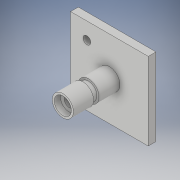
# Autodesk Inventor part: pieza_2_vinculacion
Saved by Autodesk Inventor 2019 (Build 230136000, 136)
## iProperties
Created: 2020-01-09
Part Number: pieza_2_vinculacion
Material: Generic
Document SubType Name: Modeling
Designer: Laptop
Density: 1 g/cm^3
Appearance: Default
Author: Laptop
## iProperties of the stored document pieza_2_vinculacion_3DPrint.ipt
Created: 2020-01-12
Part Number: pieza_2_vinculacion_3DPrint
Material: Generic
Document SubType Name: Modeling
Designer: Laptop
Density: 1 g/cm^3
Appearance: Default
Author: Laptop
Autodesk Inventor part; units mm, degrees
ref_plane "YZ Plane" through (0, 0, 0) normal (1, 0, 0) x (0, 1, 0)
ref_plane "XZ Plane" through (0, 0, 0) normal (0, 1, 0) x (-1, 0, 0)
sketch "Boceto1" plane through (0, 0, 0) normal (0, 0, 1) x (1, 0, 0)
  circle A0 centre (0, 0) radius 6.8
  dimension "d0" = 13.6
  constraints: 1 centre point, 1 coincident
  measures "d0" diameter of A0
extrude "Extrusión1" add sketch "Boceto1" along normal blind 30
ref_plane "Plano de trabajo1" through (0, 0, 13.5) normal (0, 0, -1) x (-1, 0, 0)
sketch "Boceto2" plane through (0, 0, 13.5) normal (0, 0, -1) x (-1, 0, 0)
  circle A0 centre (0, 0) radius 5.5
  circle A1 centre (0, 0) radius 7
  dimension "d4" = 11
  dimension "d5" = 14
  constraints: 2 centre point, 2 coincident
  measures "d4" diameter of A0
  measures "d5" diameter of A1
extrude "Extrusión2" cut sketch "Boceto2" against normal blind 3.5
sketch "Boceto3" plane through (0, 0, 0) normal (0, 0, -1) x (-1, 0, 0)
  line L0 (-25, 25) -> (25, 25)
  line L1 (25, 25) -> (25, -25)
  line L2 (25, -25) -> (-25, -25)
  line L3 (-25, -25) -> (-25, 25)
  line L4 (-25, 25) -> (25, -25) construction
  line L5 (25, 25) -> (-25, -25) construction
  line L6 (25, 25) -> (15, 25)
  line L7 (15, 25) -> (15, 16.75)
  line L8 (16.95, 14.8) -> (25, 14.8)
  line L9 (25, 14.8) -> (25, 25)
  line L10 (25, -25) -> (15, -25)
  line L11 (15, -25) -> (15, -16.75)
  line L12 (16.95, -14.8) -> (25, -14.8)
  line L13 (25, -14.8) -> (25, -25)
  line L14 (-25, 25) -> (-14.8, 25)
  line L15 (-14.8, 25) -> (-14.8, 16.95)
  line L16 (-16.75, 15) -> (-25, 15)
  line L17 (-25, 15) -> (-25, 25)
  line L18 (-25, -25) -> (-15, -25)
  line L19 (-15, -25) -> (-15, -16.9397)
  line L20 (-16.75, -15) -> (-25, -15)
  line L21 (-25, -15) -> (-25, -25)
  circle A0 centre (14.5004, 14.3004) radius 2.5
  circle A1 centre (14.5004, -14.3004) radius 2.5
  circle A2 centre (-14.8, 15) radius 1.95
  circle A3 centre (-14.8, -15) radius 1.95
  point P0 (0, 0)
  dimension "d8" = 50
  dimension "d9" = 50
  dimension "d18" = 5
  dimension "d19" = 5
  dimension "d20" = 3.9
  dimension "d21" = 3.9
  dimension "d24" = 8.25
  dimension "d25" = 8.05
  dimension "d26" = 8.25
  dimension "d27" = 8.0603
  dimension "d28" = 8.25
  dimension "d29" = 8.05
  dimension "d30" = 8.25
  dimension "d31" = 8.05
  constraints: 44 end point, 10 parallel, 8 point on circle, 5 horizontal, 5 perpendicular, 4 centre point, 2 midpoint
  measures "d8" distance of L1.end L2.end
  measures "d9" distance of L0.end L1.end
  measures "d18" diameter of A0
  measures "d19" diameter of A1
  measures "d20" diameter of A2
  measures "d21" diameter of A3
  measures "d24" distance of L16.start L16.end
  measures "d25" distance of L14.end L15.end
  measures "d26" distance of L20.start L20.end
  measures "d27" distance of L18.end L19.end
  measures "d28" distance of L6.end L7.end
  measures "d29" distance of L8.start L8.end
  measures "d30" distance of L10.end L11.end
  measures "d31" distance of L12.start L12.end
extrude "Extrusión3" add sketch "Boceto3" along normal blind 5 contours L0 L15 A2 L16 L3 | L0 L7 A0 L8 L1 L12 A1 L11 L2 L19 A3 L20 L3 L16 A2 L15 | L0 L1 L8 A0 L7 | L20 A3 L19 L2 L3 | L1 L2 L11 A1 L12
sketch "Boceto4" plane through (0, 0, 13.5) normal (0, 0, -1) x (-1, 0, 0)
  point P0 (0, 0)
sketch "Boceto5" plane through (0, 0, -5) normal (0, 0, -1) x (-1, 0, 0)
  circle A0 centre (0, 0) radius 5.5 projected
  circle A1 centre (0, 0) radius 3
  dimension "d32" = 6
  constraints: 1 centre point, 1 coincident
  measures "d32" diameter of A1
extrude "Extrusión4" cut sketch "Boceto5" against normal blind 33 contours A1
sketch "Boceto6" plane through (0, 0, 30) normal (0, 0, 1) x (1, 0, 0)
  circle A0 centre (0, 0) radius 5.5
  dimension "d35" = 11
  constraints: 1 centre point, 1 coincident
  measures "d35" diameter of A0
extrude "Extrusión5" cut sketch "Boceto6" against normal blind 4
sketch "Boceto7" plane through (0, 0, -5) normal (0, 0, -1) x (-1, 0, 0)
  circle A0 centre (-14.8, -15) radius 1.95 projected
  circle A1 centre (-14.8, 15) radius 1.95 projected
  point P0 (0, 0)
extrude "Extrusión6" add sketch "Boceto7" against normal up to surface (5 mm away)
